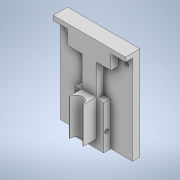
# Autodesk Inventor part: Flywheel_base
Saved by Autodesk Inventor 2021 (Build 250183000, 183)
## iProperties
Created: 2024-05-11
Part Number: Flywheel_base
Material: Generic
Document SubType Name: Modeling
Designer: Lukas
Density: 1 g/cm^3
Appearance: Default
Author: Lukas
Autodesk Inventor part; units mm, degrees
ref_plane "YZ Plane" through (0, 0, 0) normal (1, 0, 0) x (0, 1, 0)
ref_plane "XZ Plane" through (0, 0, 0) normal (0, 1, 0) x (-1, 0, 0)
ref_plane "XY Plane" through (0, 0, 0) normal (0, 0, 1) x (1, 0, 0)
sketch "Sketch1" plane through (0, 0, 0) normal (0, 0, 1) x (1, 0, 0)
  line L0 (-25, 32.5) -> (25, 32.5)
  line L1 (25, 32.5) -> (25, -32.5)
  line L2 (25, -32.5) -> (-25, -32.5)
  line L3 (-25, -32.5) -> (-25, 32.5)
  point P0 (0, 0)
  point P1 (-25, 0)
  point P2 (0, 32.5)
  dimension "d0" = 50
  dimension "d1" = 65
  constraints: 8 end point, 2 midpoint, 2 parallel, 1 horizontal, 1 horizontal alignment, 1 perpendicular, 1 vertical alignment
  measures "d0" distance of L0.start L0.end
  measures "d1" distance of L0.end L1.end
extrude "Extrusion1" add sketch "Sketch1" along normal blind 5
sketch "Sketch2" plane through (0, 0, 5) normal (0, 0, 1) x (1, 0, 0)
  line L0 (-25, -32.5) -> (25, -32.5) projected
  line L1 (25, -32.5) -> (25, 32.5) projected
  line L2 (25, 32.5) -> (-25, 32.5) projected
  line L3 (-25, 32.5) -> (-25, -32.5) projected
  line L4 (-25, 32.5) -> (-25, -32.5) projected
  line L5 (25, -32.5) -> (25, 32.5) projected
  line L6 (-25, 29.5) -> (-15, 29.5)
  line L7 (-15, 29.5) -> (-15, 19.5)
  line L8 (-15, 19.5) -> (-5, 19.5)
  line L9 (-5, 19.5) -> (-5, -2.5)
  line L10 (-5, -2.5) -> (-10, -2.5)
  line L11 (-10, -2.5) -> (-10, -32.5)
  line L12 (-10, -32.5) -> (-25, -32.5)
  line L13 (25, -32.5) -> (10, -32.5)
  line L14 (10, -32.5) -> (10, -2.5)
  line L15 (10, -2.5) -> (5, -2.5)
  line L16 (5, -2.5) -> (5, 19.5)
  line L17 (5, 19.5) -> (15, 19.5)
  line L18 (15, 19.5) -> (15, 29.5)
  line L19 (25, 29.5) -> (15, 29.5)
  circle A0 centre (-21, 23.5) radius 1.4
  circle A1 centre (21, 23.5) radius 1.4
  point P0 (0, 0)
  point P1 (15, 30)
  point P2 (-15, 30)
  dimension "d11" = 2.8
  dimension "d12" = 10
  dimension "d13" = 6
  dimension "d14" = 4
  dimension "d15" = 10
  dimension "d16" = 22
  dimension "d17" = 10
  dimension "d18" = 30
  dimension "d24" = 4
  dimension "d36" = 15
  constraints: 28 end point, 13 point on line, 9 perpendicular, 3 collinear, 2 centre point, 1 equal radius, 1 horizontal alignment, 1 vertical
  measures "d11" diameter of A0
  measures "d12" distance of L6.start L6.end
  measures "d13" distance from line of L6 A0.centre
  measures "d14" distance from line of L3 A0.centre
  measures "d15" distance of L6.end L7.end
  measures "d16" distance of L8.end L9.end
  measures "d17" distance of L7.end L8.end
  measures "d18" distance of L10.end L11.end
  measures "d24" distance from line of L1 A1.centre
  measures "d36" distance between parallel lines of L3 L11
extrude "Extrusion2" add sketch "Sketch2" along normal blind 5 contours L11 L10 L9 L8 L7 L6 L3 L2 L1 L19 L18 L17 L16 L15 L14 L0
extrude "Extrusion3" cut sketch "Sketch2" against normal through all contours A0 | A1
sketch "Sketch3" plane through (-10, -32.5, 5) normal (-1, 0, 0) x (0, 0, 1)
  circle A0 centre (3, 12) radius 1.4
  line L0 (0, 57.4) -> (0, 54.6) projected
  line L1 (-5, 65) -> (5, 65) projected
  line L2 (0, 0) -> (0, 30) projected
  point P0 (-5, 32.5)
  point P1 (0, 60)
  dimension "d25" = 53
  dimension "d26" = 3
  dimension "d27" = 2.8
  constraints: 1 centre point, 1 other
  measures "d26" distance from line of L2 A0.centre
  measures "d27" diameter of A0
extrude "Extrusion4" cut sketch "Sketch3" against normal through all
ref_plane "Work Plane1" through (-25, -26.5, 0) normal (0, -1, 0) x (1, 0, 0)
sketch "Sketch4" plane through (-25, -26.5, 0) normal (0, -1, 0) x (1, 0, 0)
  line L0 (15, 10) -> (35, 10) projected
  line L1 (20, 10) -> (20, 19)
  line L2 (20, 19) -> (20.5, 19)
  line L3 (30, 10) -> (30, 19)
  line L4 (30, 19) -> (29.5, 19)
  arc A0 (20.5, 19) -> (29.5, 19) centre (25, 19) ccw
  line L5 (50, 10) -> (0, 10) projected
  point P0 (25, 0)
  point P1 (25, 10)
  dimension "d31" = 9
  dimension "d32" = 4.5
  dimension "d33" = 0.5
  constraints: 8 end point, 3 perpendicular, 3 point on line, 2 horizontal alignment, 2 point on circle, 1 centre point, 1 collinear, 1 midpoint, 1 vertical, 1 vertical alignment
  measures "d31" distance from line of L0 A0.centre
  measures "d32" radius of A0
  measures "d33" distance of L1.end L2.end
extrude "Extrusion5" add sketch "Sketch4" against normal blind 25
equation "\"d24\" = d14"
body "Solid1"
